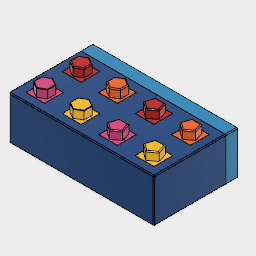
Base (Autodesk Fusion 360 design; units mm, degrees)
part number: Base
Autodesk Fusion 360 part; units mm, degrees
note: some values were not read from the file. Chosen so that the rebuilt part matches the saved one: which face or edge a step refers to.
sketch "Sketch1" plane through (0, 0, 0) normal (0, 1, 0) x (1, 0, 0) in component "Brick (1)"
  line L0 (15.9, -7.9) -> (-15.9, -7.9)
  line L1 (-15.9, -7.9) -> (-15.9, 7.9)
  line L2 (-15.9, 7.9) -> (15.9, 7.9)
  line L3 (15.9, 7.9) -> (15.9, -7.9)
  line L4 (15.9, -7.9) -> (-15.9, 7.9) construction
  line L5 (-15.9, -7.9) -> (15.9, 7.9) construction
  dimension "d53_2" = 15.8
  dimension "d54_2" = 31.8
  measures "d53_2" distance of L0.end L1.end
  measures "d54_2" distance of L1.end L2.end
extrude "Extrude6" add sketch "Sketch1" along normal blind 9.6 makes body 1 in component "Brick (1)"
sketch "Sketch2" plane through (0, 9.6, 0) normal (0, 1, 0) x (-1, 0, 0) in component "Brick (1)"
  line L0 (-15.9, -7.9) -> (15.9, -7.9)
  line L1 (15.9, -7.9) -> (15.9, 7.9)
  line L2 (15.9, 7.9) -> (-15.9, 7.9)
  line L3 (-15.9, 7.9) -> (-15.9, -7.9)
  line L4 (9.95, -1.95) -> (14.05, -1.95)
  line L5 (14.05, -1.95) -> (14.05, -6.05)
  line L6 (14.05, -6.05) -> (9.95, -6.05)
  line L7 (9.95, -6.05) -> (9.95, -1.95)
  line L8 (9.95, -1.95) -> (14.05, -6.05) construction
  line L9 (14.05, -1.95) -> (9.95, -6.05) construction
  point P0 (12, -4)
  dimension "d57_2" = 3.9
  dimension "d58_2" = 3.9
  dimension "d59_2" = 4.1
  dimension "d60_2" = 4.1
  measures "d57_2" distance of L0 P0
  measures "d58_2" distance of L1 P0
  measures "d59_2" distance of L5.end L6.end
  measures "d60_2" distance of L4.end L5.end
extrude "Extrude7" cut sketch "Sketch2" against normal blind 0.5 contours L4 L5 L6 L7 bodies 1 in component "Brick (1)"
pattern_linear "R-Pattern3" count 4 spacing 8 along (1, 0, 0) count 2 spacing 8 along (0, 0, 1) of "Extrude7" in component "Brick (1)"
fillet "Fillet1" radius 0.2 10 edges at (0, 0, -7.9) (15.9, 0, 0) (15.9, 4.8, -7.9) (0, 9.6, -7.9) (15.9, 9.6, 0) (0, 9.6, 7.9) (15.9, 4.8, 7.9) (-15.9, 4.8, 7.9) (-15.9, 0, 0) (0, 0, 7.9) on bodies 1 in component "Brick (1)"
ref_plane "WorkPlane1" through (-0.1, 4.8, -5.1) normal (0, 0, -1) x (-1, 0, 0)
split "Split2" by plane through (-0.1, 4.8, -5.1) normal (0, 0, -1) bodies 1 makes body 2 at (5.1667, 6.3333, -7.9) in component "Brick (1)"
sketch "Sketch1 (2)" plane through (0, 0, -7.9) normal (0, 0, -1) x (-1, 0, 0)
  line L0 (-15.7, 0.2) -> (15.9, 0.2)
  line L1 (15.9, 0.2) -> (15.9, 9.4)
  line L2 (15.9, 9.4) -> (-15.7, 9.4)
  line L3 (-15.7, 9.4) -> (-15.7, 0.2)
  line L4 (-15.7, 4.8) -> (15.9, 4.8) construction
  line L5 (-9.9, 2.8) -> (-13.9, 2.8)
  line L6 (-13.9, 2.8) -> (-13.9, 6.8)
  line L7 (-13.9, 6.8) -> (-9.9, 6.8)
  line L8 (-9.9, 6.8) -> (-9.9, 2.8)
  line L9 (-9.9, 2.8) -> (-13.9, 6.8) construction
  line L10 (-13.9, 2.8) -> (-9.9, 6.8) construction
  point P0 (-11.9, 4.8)
  dimension "d19" = 4
  dimension "d20" = 4
  dimension "d21" = 3.8
  measures "d19" distance of L6.end L7.end
  measures "d20" distance of L5.end L6.end
  measures "d21" distance of L4.start P0
extrude "Extrude9" add sketch "Sketch1 (2)" along normal blind 1.8 contours L5 L6 L7 L8 bodies 2 in component "Brick (1)"
pattern_linear "R-Pattern5" count 4 spacing 8 along (-1, 0, 0) of "Extrude9" in component "Brick (1)"
sketch "Sketch2 (2)" plane through (0, 0, -9.7) normal (0, 0, -1) x (-1, 0, 0)
  line L0 (-9.9, 6.8) -> (-13.9, 6.8)
  line L1 (-13.9, 6.8) -> (-13.9, 2.8)
  line L2 (-13.9, 2.8) -> (-9.9, 2.8)
  line L3 (-9.9, 2.8) -> (-9.9, 6.8)
  line L4 (-13.9, 4.8) -> (-9.9, 4.8) construction
  line L5 (-11.9, 6.8) -> (-11.9, 2.8) construction
  circle A0 centre (-11.9, 4.8) radius 1.7
  circle A1 centre (-11.9, 4.8) radius 1.2
  dimension "d28" = 3.4
  dimension "d29" = 2.4
  measures "d28" diameter of A0
  measures "d29" diameter of A1
extrude "Extrude10" cut sketch "Sketch2 (2)" against normal blind 1.8 contours A0 bodies 2 in component "Brick (1)"
extrude "Extrude11" cut 1 faces at (12.1591, 5.1553, -9.7) along direction (0, 0, 1) blind 0.2 on bodies 2 bodies 2 in component "Brick (1)"
extrude "Extrude12" cut 1 faces at (10.373, 4.7155, -7.9) along direction (0, 0, 1) blind 1 on bodies 2 bodies 2 in component "Brick (1)"
extrude "Extrude13" cut 1 faces at (12.1591, 5.1553, -9.5) along direction (0, 0, 1) blind 0.2 on bodies 2 bodies 2 in component "Brick (1)"
sketch "Sketch3" plane through (0, 0, -9.7) normal (0, 0, -1) x (-1, 0, 0)
  line L0 (-1.9, 6.8) -> (-5.9, 6.8)
  line L1 (-5.9, 6.8) -> (-5.9, 2.8)
  line L2 (-5.9, 2.8) -> (-1.9, 2.8)
  line L3 (-1.9, 2.8) -> (-1.9, 6.8)
  line L4 (-3.9, 6.8) -> (-3.9, 2.8) construction
  line L5 (-5.9, 4.8) -> (-1.9, 4.8) construction
  line L6 (-2.3, 3.2) -> (-5.5, 3.2)
  line L7 (-5.5, 3.2) -> (-5.5, 6.4)
  line L8 (-5.5, 6.4) -> (-2.3, 6.4)
  line L9 (-2.3, 6.4) -> (-2.3, 3.2)
  line L10 (-2.3, 3.2) -> (-5.5, 6.4) construction
  line L11 (-5.5, 3.2) -> (-2.3, 6.4) construction
  line L12 (-2.8, 3.7) -> (-5, 3.7)
  line L13 (-5, 3.7) -> (-5, 5.9)
  line L14 (-5, 5.9) -> (-2.8, 5.9)
  line L15 (-2.8, 5.9) -> (-2.8, 3.7)
  line L16 (-2.8, 3.7) -> (-5, 5.9) construction
  line L17 (-5, 3.7) -> (-2.8, 5.9) construction
  point P0 (-3.9, 4.8)
  point P1 (-3.9, 4.8)
  dimension "d38" = 3.2
  dimension "d39" = 3.2
  dimension "d40" = 2.2
  dimension "d41" = 2.2
  measures "d38" distance of L7.end L8.end
  measures "d39" distance of L6.end L7.end
  measures "d40" distance of L13.end L14.end
  measures "d41" distance of L12.end L13.end
extrude "Extrude14" cut sketch "Sketch3" against normal blind 2.8 contours L6 L7 L8 L9 bodies 2 in component "Brick (1)"
extrude "Extrude15" cut 1 faces at (4.2667, 5.1667, -9.7) along direction (0, 0, 1) blind 0.4 on bodies 2 bodies 2 in component "Brick (1)"
sketch "Sketch4" plane through (0, 0, -9.7) normal (0, 0, -1) x (-1, 0, 0)
  line L0 (6.1, 6.8) -> (2.1, 6.8)
  line L1 (2.1, 6.8) -> (2.1, 2.8)
  line L2 (2.1, 2.8) -> (6.1, 2.8)
  line L3 (6.1, 2.8) -> (6.1, 6.8)
  line L4 (4.1, 6.8) -> (4.1, 2.8) construction
  line L5 (2.1, 4.8) -> (6.1, 4.8) construction
  line L6 (4.1, 6.3311) -> (2.35, 3.3)
  line L7 (2.35, 3.3) -> (5.85, 3.3)
  line L8 (5.85, 3.3) -> (4.1, 6.3311)
  line L9 (4.1, 6.3311) -> (7.6, 6.3311) construction
  line L10 (4.984, 3.8) -> (4.1, 5.3311)
  line L11 (4.1, 5.3311) -> (3.216, 3.8)
  line L12 (3.216, 3.8) -> (4.984, 3.8)
  point P0 (4.1, 4.3104)
  dimension "d46" = 3.5
  dimension "d47" = 120
  dimension "d48" = 0.5
  dimension "d49" = 0.5
  measures "d46" distance of L6.start L6.end
  measures "d47" angle of L6 L9
  measures "d48" distance of L2 L7
extrude "Extrude16" cut sketch "Sketch4" against normal blind 2.8 contours L6 L7 L8 bodies 2 in component "Brick (1)"
extrude "Extrude17" cut 1 faces at (-4.1, 4.3104, -9.7) along direction (0, 0, 1) blind 0.4 on bodies 2 bodies 2 in component "Brick (1)"
sketch "Sketch5" plane through (0, 0, -9.7) normal (0, 0, -1) x (-1, 0, 0)
  line L0 (14.1, 6.8) -> (10.1, 6.8)
  line L1 (10.1, 6.8) -> (10.1, 2.8)
  line L2 (10.1, 2.8) -> (14.1, 2.8)
  line L3 (14.1, 2.8) -> (14.1, 6.8)
  line L4 (12.1, 6.8) -> (12.1, 2.8) construction
  line L5 (10.1, 4.8) -> (14.1, 4.8) construction
  circle A0 centre (12.1, 4.8) radius 1.7
  line L6 (10.4, 4.8) -> (13.8, 4.8)
  line L7 (13.8, 4.8) -> (13.8, 3.1)
  line L8 (13.8, 3.1) -> (10.4, 3.1)
  line L9 (10.4, 3.1) -> (10.4, 4.8)
  circle A1 centre (12.1, 4.8) radius 1.2
  line L10 (10.9, 4.8) -> (13.3, 4.8)
  line L11 (13.3, 4.8) -> (13.3, 3.6)
  line L12 (13.3, 3.6) -> (10.9, 3.6)
  line L13 (10.9, 3.6) -> (10.9, 4.8)
  dimension "d68" = 3.4
  dimension "d69" = 3.4
  dimension "d70" = 1.7
  dimension "d71" = 2.4
  dimension "d72" = 2.4
  dimension "d73" = 1.2
  measures "d68" diameter of A0
  measures "d69" distance of L6.start L6.end
  measures "d70" distance of L6.start L8.end
  measures "d71" diameter of A1
  measures "d72" distance of L10.start L10.end
  measures "d73" distance of L10.start L12.end
extrude "Extrude18" cut sketch "Sketch5" against normal blind 2.8 contours A0 L6 A1 | A0 L7 L8 | A0 L6 L11 L12 L13 | A0 L8 L9 bodies 2 in component "Brick (1)"
extrude "Extrude19" cut 1 faces at (-11.7, 4.4, -9.7) along direction (0, 0, 1) blind 0.4 on bodies 2 bodies 2 in component "Brick (1)"
sketch "Sketch1 (3)" plane through (0, 9.1, 0) normal (0, 1, 0) x (-1, 0, 0) in component "Stud - pentagon"
  line L0 (9.95, 1.95) -> (14.05, 1.95)
  line L1 (14.05, 1.95) -> (14.05, 6.05)
  line L2 (14.05, 6.05) -> (9.95, 6.05)
  line L3 (9.95, 6.05) -> (9.95, 1.95)
  line L4 (9.95, 6.05) -> (14.05, 6.05)
  line L5 (14.05, 6.05) -> (14.05, 1.95)
  line L6 (14.05, 1.95) -> (9.95, 1.95)
  line L7 (9.95, 1.95) -> (9.95, 6.05)
  line L8 (9.95, 6.05) -> (14.05, 1.95) construction
  line L9 (14.05, 6.05) -> (9.95, 1.95) construction
  line L10 (15.9, -7.9) -> (15.9, 7.9)
  point P0 (12, 4)
extrude "Extrude1" add sketch "Sketch1 (3)" along normal blind 0.5 separate body makes body 3 in component "Stud - pentagon"
sketch "Sketch3 (2)" plane through (0, 9.6, 0) normal (0, 1, 0) x (-1, 0, 0) in component "Stud - pentagon"
  line L0 (9.95, 1.95) -> (14.05, 1.95)
  line L1 (14.05, 1.95) -> (14.05, 6.05)
  line L2 (14.05, 6.05) -> (9.95, 6.05)
  line L3 (9.95, 6.05) -> (9.95, 1.95)
  line L4 (12, 5.8) -> (10.2881, 4.5562)
  line L5 (10.2881, 4.5562) -> (10.942, 2.5438)
  line L6 (10.942, 2.5438) -> (13.058, 2.5438)
  line L7 (13.058, 2.5438) -> (13.7119, 4.5562)
  line L8 (13.7119, 4.5562) -> (12, 5.8)
  line L9 (14.05, 4) -> (9.5225, 4) construction
  line L10 (12, 1.95) -> (12, 6.05) construction
  point P0 (12, 4)
  dimension "d155_1" = 1.8
  measures "d155_1" distance of L4.start P0
extrude "Extrude3" add sketch "Sketch3 (2)" along normal blind 1.8 contours L4 L5 L6 L7 L8 bodies 3 in component "Stud - pentagon"
fillet "Fillet1'" radius 0.2 5 edges at (-12.856, 11.4, 5.1781) (-13.385, 11.4, 3.55) (-12, 11.4, 2.5438) (-10.615, 11.4, 3.55) (-11.144, 11.4, 5.1781) on bodies 3 in component "Stud - pentagon"
sketch "Sketch1 (4)" plane through (0, 9.1, 0) normal (0, 1, 0) x (-1, 0, 0) in component "Stud - pentagon (1)"
  line L0 (9.95, 1.95) -> (14.05, 1.95)
  line L1 (14.05, 1.95) -> (14.05, 6.05)
  line L2 (14.05, 6.05) -> (9.95, 6.05)
  line L3 (9.95, 6.05) -> (9.95, 1.95)
  line L4 (9.95, 6.05) -> (14.05, 6.05)
  line L5 (14.05, 6.05) -> (14.05, 1.95)
  line L6 (14.05, 1.95) -> (9.95, 1.95)
  line L7 (9.95, 1.95) -> (9.95, 6.05)
  line L8 (9.95, 6.05) -> (14.05, 1.95) construction
  line L9 (14.05, 6.05) -> (9.95, 1.95) construction
  line L10 (15.9, -7.9) -> (15.9, 7.9)
  point P0 (12, 4)
extrude "Extrude1'" add sketch "Sketch1 (4)" along normal blind 0.5 separate body makes body 4 in component "Stud - pentagon (1)"
sketch "Sketch3 (3)" plane through (0, 9.6, 0) normal (0, 1, 0) x (-1, 0, 0) in component "Stud - pentagon (1)"
  line L0 (9.95, 1.95) -> (14.05, 1.95)
  line L1 (14.05, 1.95) -> (14.05, 6.05)
  line L2 (14.05, 6.05) -> (9.95, 6.05)
  line L3 (9.95, 6.05) -> (9.95, 1.95)
  line L4 (12, 5.8) -> (10.2881, 4.5562)
  line L5 (10.2881, 4.5562) -> (10.942, 2.5438)
  line L6 (10.942, 2.5438) -> (13.058, 2.5438)
  line L7 (13.058, 2.5438) -> (13.7119, 4.5562)
  line L8 (13.7119, 4.5562) -> (12, 5.8)
  line L9 (14.05, 4) -> (9.5225, 4) construction
  line L10 (12, 1.95) -> (12, 6.05) construction
  point P0 (12, 4)
  dimension "d155_2" = 1.8
  measures "d155_2" distance of L4.start P0
extrude "Extrude3'" add sketch "Sketch3 (3)" along normal blind 1.8 contours L4 L5 L6 L7 L8 bodies 4 in component "Stud - pentagon (1)"
fillet "Fillet1''" radius 0.2 5 edges at (-12.856, 11.4, 5.1781) (-13.385, 11.4, 3.55) (-12, 11.4, 2.5438) (-10.615, 11.4, 3.55) (-11.144, 11.4, 5.1781) on bodies 4 in component "Stud - pentagon (1)"
sketch "Sketch1 (5)" plane through (0, 9.1, 0) normal (0, 1, 0) x (-1, 0, 0) in component "Stud - hexagon"
  line L0 (9.95, -6.05) -> (14.05, -6.05)
  line L1 (14.05, -6.05) -> (14.05, -1.95)
  line L2 (14.05, -1.95) -> (9.95, -1.95)
  line L3 (9.95, -1.95) -> (9.95, -6.05)
  line L4 (9.95, -1.95) -> (14.05, -1.95)
  line L5 (14.05, -1.95) -> (14.05, -6.05)
  line L6 (14.05, -6.05) -> (9.95, -6.05)
  line L7 (9.95, -6.05) -> (9.95, -1.95)
  line L8 (9.95, -1.95) -> (14.05, -6.05) construction
  line L9 (14.05, -1.95) -> (9.95, -6.05) construction
  point P0 (12, -4)
extrude "Extrude1''" add sketch "Sketch1 (5)" along normal blind 0.5 separate body makes body 5 in component "Stud - hexagon"
sketch "Sketch4 (2)" plane through (0, 9.6, 0) normal (0, 1, 0) x (-1, 0, 0) in component "Stud - hexagon"
  line L0 (9.95, -6.05) -> (14.05, -6.05)
  line L1 (14.05, -6.05) -> (14.05, -1.95)
  line L2 (14.05, -1.95) -> (9.95, -1.95)
  line L3 (9.95, -1.95) -> (9.95, -6.05)
  line L4 (10.4412, -3.1) -> (10.4412, -4.9)
  line L5 (10.4412, -4.9) -> (12, -5.8)
  line L6 (12, -5.8) -> (13.5588, -4.9)
  line L7 (13.5588, -4.9) -> (13.5588, -3.1)
  line L8 (13.5588, -3.1) -> (12, -2.2)
  line L9 (12, -2.2) -> (10.4412, -3.1)
  line L10 (12, -6.05) -> (12, -2.2) construction
  line L11 (14.05, -4) -> (9.95, -4) construction
  point P0 (12, -4)
  dimension "d158_1" = 1.8
  measures "d158_1" distance of L4.start P0
extrude "Extrude3''" add sketch "Sketch4 (2)" along normal blind 1.8 contours L4 L5 L6 L7 L8 L9 bodies 5 in component "Stud - hexagon"
fillet "Fillet1'''" radius 0.2 6 edges at (-11.2206, 11.4, -5.35) (-10.4412, 11.4, -4) (-11.2206, 11.4, -2.65) (-12.7794, 11.4, -2.65) (-13.5588, 11.4, -4) (-12.7794, 11.4, -5.35) on bodies 5 in component "Stud - hexagon"
sketch "Sketch1 (6)" plane through (0, 9.1, 0) normal (0, 1, 0) x (-1, 0, 0) in component "Stud - hexagon (1)"
  line L0 (9.95, -6.05) -> (14.05, -6.05)
  line L1 (14.05, -6.05) -> (14.05, -1.95)
  line L2 (14.05, -1.95) -> (9.95, -1.95)
  line L3 (9.95, -1.95) -> (9.95, -6.05)
  line L4 (9.95, -1.95) -> (14.05, -1.95)
  line L5 (14.05, -1.95) -> (14.05, -6.05)
  line L6 (14.05, -6.05) -> (9.95, -6.05)
  line L7 (9.95, -6.05) -> (9.95, -1.95)
  line L8 (9.95, -1.95) -> (14.05, -6.05) construction
  line L9 (14.05, -1.95) -> (9.95, -6.05) construction
  point P0 (12, -4)
extrude "Extrude1'''" add sketch "Sketch1 (6)" along normal blind 0.5 separate body makes body 6 in component "Stud - hexagon (1)"
sketch "Sketch4 (3)" plane through (0, 9.6, 0) normal (0, 1, 0) x (-1, 0, 0) in component "Stud - hexagon (1)"
  line L0 (9.95, -6.05) -> (14.05, -6.05)
  line L1 (14.05, -6.05) -> (14.05, -1.95)
  line L2 (14.05, -1.95) -> (9.95, -1.95)
  line L3 (9.95, -1.95) -> (9.95, -6.05)
  line L4 (10.4412, -3.1) -> (10.4412, -4.9)
  line L5 (10.4412, -4.9) -> (12, -5.8)
  line L6 (12, -5.8) -> (13.5588, -4.9)
  line L7 (13.5588, -4.9) -> (13.5588, -3.1)
  line L8 (13.5588, -3.1) -> (12, -2.2)
  line L9 (12, -2.2) -> (10.4412, -3.1)
  line L10 (12, -6.05) -> (12, -2.2) construction
  line L11 (14.05, -4) -> (9.95, -4) construction
  point P0 (12, -4)
  dimension "d158_2" = 1.8
  measures "d158_2" distance of L4.start P0
extrude "Extrude3'''" add sketch "Sketch4 (3)" along normal blind 1.8 contours L4 L5 L6 L7 L8 L9 bodies 6 in component "Stud - hexagon (1)"
fillet "Fillet1''''" radius 0.1 6 edges at (-11.2206, 11.4, -5.35) (-10.4412, 11.4, -4) (-11.2206, 11.4, -2.65) (-12.7794, 11.4, -2.65) (-13.5588, 11.4, -4) (-12.7794, 11.4, -5.35) on bodies 6 in component "Stud - hexagon (1)"
fillet "Fillet2" radius 0.1 16 edges at (11.9, 6.8, -9.7) (13.9, 4.8, -9.7) (9.9, 4.8, -9.7) (11.9, 2.8, -9.7) (5.9, 4.8, -9.7) (3.9, 6.8, -9.7) (1.9, 4.8, -9.7) (3.9, 2.8, -9.7) (-2.1, 4.8, -9.7) (-4.1, 6.8, -9.7) (-6.1, 4.8, -9.7) (-4.1, 2.8, -9.7) (-10.1, 4.8, -9.7) (-12.1, 6.8, -9.7) (-14.1, 4.8, -9.7) (-12.1, 2.8, -9.7) on bodies 2 in component "Brick (1)"
fillet "Fillet3" radius 0.1 12 edges at (13.0188, 5.2339, -9.3) (3.9, 5.9, -9.3) (5, 4.8, -9.3) (3.9, 3.7, -9.3) (2.8, 4.8, -9.3) (-3.658, 4.5655, -9.3) (-4.542, 4.5655, -9.3) (-4.1, 3.8, -9.3) (-10.9, 4.2, -9.3) (-12.1, 6, -9.3) (-13.3, 4.2, -9.3) (-12.1, 3.6, -9.3) on bodies 2 in component "Brick (1)"
sketch "Sketch1 (7)" plane through (0, 9.1, 0) normal (0, 1, 0) x (-1, 0, 0) in component "Stud - pentagon (1) (1)"
  line L0 (9.95, 1.95) -> (14.05, 1.95)
  line L1 (14.05, 1.95) -> (14.05, 6.05)
  line L2 (14.05, 6.05) -> (9.95, 6.05)
  line L3 (9.95, 6.05) -> (9.95, 1.95)
  line L4 (9.95, 6.05) -> (14.05, 6.05)
  line L5 (14.05, 6.05) -> (14.05, 1.95)
  line L6 (14.05, 1.95) -> (9.95, 1.95)
  line L7 (9.95, 1.95) -> (9.95, 6.05)
  line L8 (9.95, 6.05) -> (14.05, 1.95) construction
  line L9 (14.05, 6.05) -> (9.95, 1.95) construction
  line L10 (15.9, -7.9) -> (15.9, 7.9)
  point P0 (12, 4)
extrude "Extrude1''''" add sketch "Sketch1 (7)" along normal blind 0.5 separate body makes body 7 in component "Stud - pentagon (1) (1)"
sketch "Sketch3 (4)" plane through (0, 9.6, 0) normal (0, 1, 0) x (-1, 0, 0) in component "Stud - pentagon (1) (1)"
  line L0 (9.95, 1.95) -> (14.05, 1.95)
  line L1 (14.05, 1.95) -> (14.05, 6.05)
  line L2 (14.05, 6.05) -> (9.95, 6.05)
  line L3 (9.95, 6.05) -> (9.95, 1.95)
  line L4 (12, 5.8) -> (10.2881, 4.5562)
  line L5 (10.2881, 4.5562) -> (10.942, 2.5438)
  line L6 (10.942, 2.5438) -> (13.058, 2.5438)
  line L7 (13.058, 2.5438) -> (13.7119, 4.5562)
  line L8 (13.7119, 4.5562) -> (12, 5.8)
  line L9 (14.05, 4) -> (9.5225, 4) construction
  line L10 (12, 1.95) -> (12, 6.05) construction
  point P0 (12, 4)
  dimension "d155_2_1" = 1.8
  measures "d155_2_1" distance of L4.start P0
extrude "Extrude3''''" add sketch "Sketch3 (4)" along normal blind 1.8 contours L4 L5 L6 L7 L8 bodies 7 in component "Stud - pentagon (1) (1)"
fillet "Fillet1'''''" radius 0.2 5 edges at (-12.856, 11.4, 5.1781) (-13.385, 11.4, 3.55) (-12, 11.4, 2.5438) (-10.615, 11.4, 3.55) (-11.144, 11.4, 5.1781) on bodies 7 in component "Stud - pentagon (1) (1)"
sketch "Sketch1 (8)" plane through (0, 9.1, 0) normal (0, 1, 0) x (-1, 0, 0) in component "Stud - pentagon (1) (1) (1)"
  line L0 (9.95, 1.95) -> (14.05, 1.95)
  line L1 (14.05, 1.95) -> (14.05, 6.05)
  line L2 (14.05, 6.05) -> (9.95, 6.05)
  line L3 (9.95, 6.05) -> (9.95, 1.95)
  line L4 (9.95, 6.05) -> (14.05, 6.05)
  line L5 (14.05, 6.05) -> (14.05, 1.95)
  line L6 (14.05, 1.95) -> (9.95, 1.95)
  line L7 (9.95, 1.95) -> (9.95, 6.05)
  line L8 (9.95, 6.05) -> (14.05, 1.95) construction
  line L9 (14.05, 6.05) -> (9.95, 1.95) construction
  line L10 (15.9, -7.9) -> (15.9, 7.9)
  point P0 (12, 4)
extrude "Extrude1'''''" add sketch "Sketch1 (8)" along normal blind 0.5 separate body makes body 8 in component "Stud - pentagon (1) (1) (1)"
sketch "Sketch3 (5)" plane through (0, 9.6, 0) normal (0, 1, 0) x (-1, 0, 0) in component "Stud - pentagon (1) (1) (1)"
  line L0 (9.95, 1.95) -> (14.05, 1.95)
  line L1 (14.05, 1.95) -> (14.05, 6.05)
  line L2 (14.05, 6.05) -> (9.95, 6.05)
  line L3 (9.95, 6.05) -> (9.95, 1.95)
  line L4 (12, 5.8) -> (10.2881, 4.5562)
  line L5 (10.2881, 4.5562) -> (10.942, 2.5438)
  line L6 (10.942, 2.5438) -> (13.058, 2.5438)
  line L7 (13.058, 2.5438) -> (13.7119, 4.5562)
  line L8 (13.7119, 4.5562) -> (12, 5.8)
  line L9 (14.05, 4) -> (9.5225, 4) construction
  line L10 (12, 1.95) -> (12, 6.05) construction
  point P0 (12, 4)
  dimension "d155_2_1_1" = 1.8
  measures "d155_2_1_1" distance of L4.start P0
extrude "Extrude3'''''" add sketch "Sketch3 (5)" along normal blind 1.8 contours L4 L5 L6 L7 L8 bodies 8 in component "Stud - pentagon (1) (1) (1)"
fillet "Fillet1''''''" radius 0.2 5 edges at (-12.856, 11.4, 5.1781) (-13.385, 11.4, 3.55) (-12, 11.4, 2.5438) (-10.615, 11.4, 3.55) (-11.144, 11.4, 5.1781) on bodies 8 in component "Stud - pentagon (1) (1) (1)"
sketch "Sketch1 (9)" plane through (0, 9.1, 0) normal (0, 1, 0) x (-1, 0, 0) in component "Stud - hexagon (2)"
  line L0 (9.95, -6.05) -> (14.05, -6.05)
  line L1 (14.05, -6.05) -> (14.05, -1.95)
  line L2 (14.05, -1.95) -> (9.95, -1.95)
  line L3 (9.95, -1.95) -> (9.95, -6.05)
  line L4 (9.95, -1.95) -> (14.05, -1.95)
  line L5 (14.05, -1.95) -> (14.05, -6.05)
  line L6 (14.05, -6.05) -> (9.95, -6.05)
  line L7 (9.95, -6.05) -> (9.95, -1.95)
  line L8 (9.95, -1.95) -> (14.05, -6.05) construction
  line L9 (14.05, -1.95) -> (9.95, -6.05) construction
  point P0 (12, -4)
extrude "Extrude1''''''" add sketch "Sketch1 (9)" along normal blind 0.5 separate body makes body 9 in component "Stud - hexagon (2)"
sketch "Sketch4 (4)" plane through (0, 9.6, 0) normal (0, 1, 0) x (-1, 0, 0) in component "Stud - hexagon (2)"
  line L0 (9.95, -6.05) -> (14.05, -6.05)
  line L1 (14.05, -6.05) -> (14.05, -1.95)
  line L2 (14.05, -1.95) -> (9.95, -1.95)
  line L3 (9.95, -1.95) -> (9.95, -6.05)
  line L4 (10.4412, -3.1) -> (10.4412, -4.9)
  line L5 (10.4412, -4.9) -> (12, -5.8)
  line L6 (12, -5.8) -> (13.5588, -4.9)
  line L7 (13.5588, -4.9) -> (13.5588, -3.1)
  line L8 (13.5588, -3.1) -> (12, -2.2)
  line L9 (12, -2.2) -> (10.4412, -3.1)
  line L10 (12, -6.05) -> (12, -2.2) construction
  line L11 (14.05, -4) -> (9.95, -4) construction
  point P0 (12, -4)
  dimension "d158_1_1" = 1.8
  measures "d158_1_1" distance of L4.start P0
extrude "Extrude3''''''" add sketch "Sketch4 (4)" along normal blind 1.8 contours L4 L5 L6 L7 L8 L9 bodies 9 in component "Stud - hexagon (2)"
fillet "Fillet1'''''''" radius 0.2 6 edges at (-11.2206, 11.4, -5.35) (-10.4412, 11.4, -4) (-11.2206, 11.4, -2.65) (-12.7794, 11.4, -2.65) (-13.5588, 11.4, -4) (-12.7794, 11.4, -5.35) on bodies 9 in component "Stud - hexagon (2)"
sketch "Sketch1 (10)" plane through (0, 9.1, 0) normal (0, 1, 0) x (-1, 0, 0) in component "Stud - hexagon (1) (1)"
  line L0 (9.95, -6.05) -> (14.05, -6.05)
  line L1 (14.05, -6.05) -> (14.05, -1.95)
  line L2 (14.05, -1.95) -> (9.95, -1.95)
  line L3 (9.95, -1.95) -> (9.95, -6.05)
  line L4 (9.95, -1.95) -> (14.05, -1.95)
  line L5 (14.05, -1.95) -> (14.05, -6.05)
  line L6 (14.05, -6.05) -> (9.95, -6.05)
  line L7 (9.95, -6.05) -> (9.95, -1.95)
  line L8 (9.95, -1.95) -> (14.05, -6.05) construction
  line L9 (14.05, -1.95) -> (9.95, -6.05) construction
  point P0 (12, -4)
extrude "Extrude1'''''''" add sketch "Sketch1 (10)" along normal blind 0.5 separate body makes body 10 in component "Stud - hexagon (1) (1)"
sketch "Sketch4 (5)" plane through (0, 9.6, 0) normal (0, 1, 0) x (-1, 0, 0) in component "Stud - hexagon (1) (1)"
  line L0 (9.95, -6.05) -> (14.05, -6.05)
  line L1 (14.05, -6.05) -> (14.05, -1.95)
  line L2 (14.05, -1.95) -> (9.95, -1.95)
  line L3 (9.95, -1.95) -> (9.95, -6.05)
  line L4 (10.4412, -3.1) -> (10.4412, -4.9)
  line L5 (10.4412, -4.9) -> (12, -5.8)
  line L6 (12, -5.8) -> (13.5588, -4.9)
  line L7 (13.5588, -4.9) -> (13.5588, -3.1)
  line L8 (13.5588, -3.1) -> (12, -2.2)
  line L9 (12, -2.2) -> (10.4412, -3.1)
  line L10 (12, -6.05) -> (12, -2.2) construction
  line L11 (14.05, -4) -> (9.95, -4) construction
  point P0 (12, -4)
  dimension "d158_2_1" = 1.8
  measures "d158_2_1" distance of L4.start P0
extrude "Extrude3'''''''" add sketch "Sketch4 (5)" along normal blind 1.8 contours L4 L5 L6 L7 L8 L9 bodies 10 in component "Stud - hexagon (1) (1)"
fillet "Fillet1''''''''" radius 0.1 6 edges at (-11.2206, 11.4, -5.35) (-10.4412, 11.4, -4) (-11.2206, 11.4, -2.65) (-12.7794, 11.4, -2.65) (-13.5588, 11.4, -4) (-12.7794, 11.4, -5.35) on bodies 10 in component "Stud - hexagon (1) (1)"
fillet "Fillet5" radius 0.1 32 edges at (13.9, 6.8, -8.75) (13.8707, 6.7707, -9.6707) (9.9, 6.8, -8.75) (9.9293, 6.7707, -9.6707) (5.9, 6.8, -8.75) (5.8707, 6.7707, -9.6707) (1.9, 6.8, -8.75) (1.9293, 6.7707, -9.6707) (-2.1, 6.8, -8.75) (-2.1293, 6.7707, -9.6707) (-6.1, 6.8, -8.75) (-6.0707, 6.7707, -9.6707) (-10.1, 6.8, -8.75) (-10.1293, 6.7707, -9.6707) (-14.1, 6.8, -8.75) (-14.0707, 6.7707, -9.6707) (13.9, 2.8, -8.75) (13.8707, 2.8293, -9.6707) (9.9, 2.8, -8.75) (9.9293, 2.8293, -9.6707) (5.9, 2.8, -8.75) (5.8707, 2.8293, -9.6707) (1.9, 2.8, -8.75) (1.9293, 2.8293, -9.6707) (-2.1, 2.8, -8.75) (-2.1293, 2.8293, -9.6707) (-6.1, 2.8, -8.75) (-6.0707, 2.8293, -9.6707) (-10.1, 2.8, -8.75) (-10.1293, 2.8293, -9.6707) (-14.1, 2.8, -8.75) (-14.0707, 2.8293, -9.6707) on bodies 2 in component "Brick (1)"
move_body "Move1" bodies 2 to x (1, 0, 0) y (0, 1, 0) z (0, 0, 1) at (0, 0, -2.8) in component "Brick (1)"
extrude "Extrude20" add 1 faces at (12.6833, 9.1, -8.2167) along direction (0, 1, 0) blind 0.5 on bodies 2 bodies 2 in component "Brick (1)"
extrude "Extrude21" add 1 faces at (4.6833, 9.1, -8.2167) along direction (0, 1, 0) blind 0.5 on bodies 2 bodies 2 in component "Brick (1)"
extrude "Extrude22" add 1 faces at (-3.3167, 9.1, -8.2167) along direction (0, 1, 0) blind 0.5 on bodies 2 bodies 2 in component "Brick (1)"
extrude "Extrude23" add 1 faces at (-11.3167, 9.1, -8.2167) along direction (0, 1, 0) blind 0.5 on bodies 2 bodies 2 in component "Brick (1)"
extrude "Extrude24" add 1 faces at (0.65, 3.0333, -5.1) along direction (0, 0, -1) blind 2.7999 on bodies 1 bodies 1 in component "Brick (1)"
sketch "Sketch6" plane through (0, 9.1, 0) normal (0, 1, 0) x (-1, 0, 0)
  line L0 (6.05, -7.8999) -> (6.05, -1.95)
  line L1 (6.05, -1.95) -> (1.95, -1.95)
  line L2 (1.95, -1.95) -> (1.95, -7.8999)
  line L3 (1.95, -7.8999) -> (6.05, -7.8999)
  line L4 (6.05, -6.05) -> (1.95, -6.05)
  point P0 (6.05, -6.05)
  point P1 (1.95, -6.05)
extrude "Extrude25" add sketch "Sketch6" along normal blind 0.5 contours L0 L2 L3 L4 bodies 1 in component "Brick (1)"
sketch "Sketch7" plane through (0, 9.1, 0) normal (0, 1, 0) x (-1, 0, 0)
  line L0 (14.05, -7.8999) -> (14.05, -1.95)
  line L1 (14.05, -1.95) -> (9.95, -1.95)
  line L2 (9.95, -1.95) -> (9.95, -7.8999)
  line L3 (9.95, -7.8999) -> (14.05, -7.8999)
  line L4 (14.05, -6.05) -> (9.95, -6.05)
  point P0 (14.05, -6.05)
  point P1 (9.95, -6.05)
extrude "Extrude26" add sketch "Sketch7" along normal blind 0.5 contours L0 L2 L3 L4 bodies 1 in component "Brick (1)"
sketch "Sketch8" plane through (0, 9.1, 0) normal (0, 1, 0) x (-1, 0, 0)
  line L0 (-1.95, -7.8999) -> (-1.95, -1.95)
  line L1 (-1.95, -1.95) -> (-6.05, -1.95)
  line L2 (-6.05, -1.95) -> (-6.05, -7.8999)
  line L3 (-6.05, -7.8999) -> (-1.95, -7.8999)
  line L4 (-1.95, -6.05) -> (-6.05, -6.05)
  point P0 (-1.95, -6.05)
  point P1 (-6.05, -6.05)
extrude "Extrude27" add sketch "Sketch8" along normal blind 0.5 contours L0 L2 L3 L4 bodies 1 in component "Brick (1)"
sketch "Sketch9" plane through (0, 9.1, 0) normal (0, 1, 0) x (-1, 0, 0)
  line L0 (-9.95, -7.8999) -> (-9.95, -1.95)
  line L1 (-9.95, -1.95) -> (-14.05, -1.95)
  line L2 (-14.05, -1.95) -> (-14.05, -7.8999)
  line L3 (-14.05, -7.8999) -> (-9.95, -7.8999)
  line L4 (-9.95, -6.05) -> (-14.05, -6.05)
  point P0 (-9.95, -6.05)
  point P1 (-14.05, -6.05)
extrude "Extrude28" add sketch "Sketch9" along normal blind 0.5 contours L0 L2 L3 L4 bodies 1 in component "Brick (1)"
component "Brick (1)" placed x (1, 0, 0) y (0, 1, 0) z (0, 0, 1) at (0, 0, 0)
component "Stud - pentagon (1)" placed x (1, 0, 0) y (0, 1, 0) z (0, 0, 1) at (24, 0, -8) in component "Brick (1)"
component "Stud - hexagon" placed x (1, 0, 0) y (0, 1, 0) z (0, 0, 1) at (8, 0, 0) in component "Brick (1)"
component "Stud - hexagon (1)" placed x (1, 0, 0) y (0, 1, 0) z (0, 0, 1) at (8, 0, 8) in component "Brick (1)"
component "Stud - pentagon (1) (1)" placed x (1, 0, 0) y (0, 1, 0) z (0, 0, 1) at (16, 0, -8) in component "Brick (1)"
component "Stud - pentagon (1) (1) (1)" placed x (1, 0, 0) y (0, 1, 0) z (0, 0, 1) at (16, 0, 0) in component "Brick (1)"
component "Stud - hexagon (2)" placed x (1, 0, 0) y (0, 1, 0) z (0, 0, 1) at (0, 0, 0) in component "Brick (1)"
component "Stud - hexagon (1) (1)" placed x (1, 0, 0) y (0, 1, 0) z (0, 0, 1) at (0, 0, 8) in component "Brick (1)"
component "Stud - pentagon" placed x (1, 0, 0) y (0, 1, 0) z (0, 0, 1) at (24, 0, 0) in component "Brick (1)"
equation "d53_1 = width_1 * spacing_1 - gap_1"
equation "d54_1 = length_1 * spacing_1 - gap_1"
equation "d55_1 = height_1"
equation "d56_1 = 0.0 deg"
equation "d61_1 = -( thickness_1 / 2 )"
equation "d62_1 = 0.0 deg"
equation "d63_1 = length_1"
equation "d64_1 = width_1"
equation "d65_1 = spacing_1"
equation "d66_1 = spacing_1"
equation "d164_1 = 0.20 mm"
equation "d171_1 = 0.20 mm"
equation "d173_1 = 0.20 mm"
equation "d174_1 = 0.20 mm"
equation "width_1 = 2"
equation "length_1 = 4"
equation "brick_1 = 9.6 mm"
equation "height_1 = brick_1"
equation "spacing_1 = 8 mm"
equation "gap_1 = 0.2 mm"
equation "thickness_1 = 1 mm"
equation "d141_1 = thickness_2 / 2"
equation "d142_1 = 0.0 deg"
equation "d156_1 = stud_1"
equation "d157_1 = 0.0 deg"
equation "d169_1 = 0.20 mm"
equation "stud = 1.8 mm"
equation "thickness_2 = 1 mm"
equation "stud_1 = 1.8 mm"
equation "thickness_3 = 1 mm"
equation "stud_2 = 1.8 mm"
equation "d132_1 = thickness_4 / 2"
equation "d133_1 = 0.0 deg"
equation "d138_1 = stud_3"
equation "d139_1 = 0.0 deg"
equation "d167_1 = 0.20 mm"
equation "thickness_4 = 1 mm"
equation "stud_3 = 1.8 mm"
equation "thickness_5 = 1 mm"
equation "stud_4 = 1.8 mm"
equation "thickness_6 = 1 mm"
equation "stud_5 = 1.8 mm"
equation "thickness_7 = 1 mm"
equation "stud_6 = 1.8 mm"
equation "d147_1 = thickness_8 / 2"
equation "d148_1 = 0.0 deg"
equation "d159_1 = stud_7"
equation "d160_1 = 0.0 deg"
equation "d170_1 = 0.20 mm"
equation "thickness_8 = 1 mm"
equation "stud_7 = 1.8 mm"
equation "thickness_9 = 1 mm"
equation "stud_8 = 1.8 mm"
equation "d53_2 = width_2 * spacing_2 - gap_2"
equation "d54_2 = length_2 * spacing_2 - gap_2"
equation "d55_2 = height_2"
equation "d61_2 = -( thickness_10 / 2 )"
equation "d63_2 = length_2"
equation "d64_2 = width_2"
equation "d65_2 = spacing_2"
equation "d66_2 = spacing_2"
equation "width_2 = 2"
equation "length_2 = 4"
equation "brick_2 = 9.6 mm"
equation "height_2 = brick_2"
equation "spacing_2 = 8 mm"
equation "gap_2 = 0.2 mm"
equation "thickness_10 = 1 mm"
equation "d18 = -( stud + thickness_1 )"
equation "d24 = length_1"
equation "thickness_11 = 1 mm"
equation "stud_9 = 1.8 mm"
equation "thickness_12 = 1 mm"
equation "stud_10 = 1.8 mm"
equation "thickness_13 = 1 mm"
equation "stud_11 = 1.8 mm"
equation "thickness_14 = 1 mm"
equation "stud_12 = 1.8 mm"
equation "d141_1 = thickness_15 / 2"
equation "d156_1 = stud_13"
equation "thickness_15 = 1 mm"
equation "stud_13 = 1.8 mm"
equation "d141_2 = thickness_16 / 2"
equation "d156_2 = stud_14"
equation "thickness_16 = 1 mm"
equation "stud_14 = 1.8 mm"
equation "d147_1 = thickness_17 / 2"
equation "d159_1 = stud_15"
equation "thickness_17 = 1 mm"
equation "stud_15 = 1.8 mm"
equation "d147_2 = thickness_18 / 2"
equation "d159_2 = stud_16"
equation "thickness_18 = 1 mm"
equation "stud_16 = 1.8 mm"
equation "d141_2_1 = thickness_16 / 2"
equation "d156_2_1 = stud_14"
equation "d141_2_1_1 = thickness_16 / 2"
equation "d156_2_1_1 = stud_14"
equation "d147_1_1 = thickness_17 / 2"
equation "d159_1_1 = stud_15"
equation "d147_2_1 = thickness_18 / 2"
equation "d159_2_1 = stud_16"
equation "d90 = ( stud + thickness_1 ) - 0.0001 mm"
